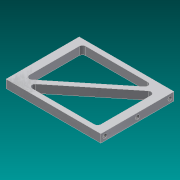
# Autodesk Inventor part: リンク_ふくらはぎ_サブフレーム_1_1(予備案)
Saved by Autodesk Inventor 2016 (Build 200138000, 138)
## iProperties
Created: 2016-06-03
Part Number: リンク_ふくらはぎ_サブフレーム_1_1(予備案)
Material: アルミニウム 2014-T4
Document SubType Name: Modeling
Designer: hiroaki
Density: 2.8 g/cm^3
Appearance: サテン
Mass: 12.9723 g
Surface Area: 43.6812 cm^2
Volume: 4.63295 cm^3
Author: hiroaki
Autodesk Inventor part; units mm, degrees
ref_plane "YZ Plane" through (0, 0, 0) normal (1, 0, 0) x (0, 1, 0)
ref_plane "XZ Plane" through (0, 0, 0) normal (0, 1, 0) x (-1, 0, 0)
ref_plane "XY Plane" through (0, 0, 0) normal (0, 0, 1) x (1, 0, 0)
sketch "スケッチ1" plane through (0, 0, 0) normal (0, 0, 1) x (1, 0, 0)
  line L0 (-29.15, 22.5) -> (29.15, 22.5)
  line L1 (29.15, 22.5) -> (29.15, -22.5)
  line L2 (29.15, -22.5) -> (-29.15, -22.5)
  line L3 (-29.15, -22.5) -> (-29.15, 22.5)
  line L4 (-24.15, 19.5) -> (24.15, 19.5) construction
  line L5 (24.15, 19.5) -> (24.15, -19.5) construction
  line L6 (24.15, -19.5) -> (-24.15, -19.5) construction
  line L7 (-24.15, -19.5) -> (-24.15, 19.5) construction
  line L8 (24.15, 19.5) -> (-24.15, -19.5) construction
  line L9 (-24.15, -17.5721) -> (-24.15, 19.5)
  line L10 (-24.15, 19.5) -> (21.7623, 19.5)
  line L11 (21.7623, 19.5) -> (-24.15, -17.5721)
  line L12 (-21.7623, -19.5) -> (24.15, -19.5)
  line L13 (24.15, -19.5) -> (24.15, 17.5721)
  line L14 (24.15, 17.5721) -> (-21.7623, -19.5)
  line L15 (-29.15, 20) -> (29.15, 20) construction
  line L16 (29.15, -20) -> (-29.15, -20) construction
  line L17 (29.15, 20) -> (29.15, -20) construction
  point P0 (0, 0)
  point P1 (0, 19.5)
  point P2 (0, 22.5)
  point P3 (24.15, 0)
  point P4 (29.15, 0)
  dimension "d0" = 5
  dimension "d1" = 3
  dimension "d2" = 1.5
  dimension "d3" = 40
  dimension "d4" = 2.5
  dimension "d19" = 58.3
  constraints: 36 end point, 6 parallel, 5 collinear, 5 horizontal, 5 midpoint, 4 perpendicular, 4 point on line, 2 horizontal alignment, 2 vertical alignment, 1 vertical, 1 other
  measures "d0" distance between parallel lines of L3 L7
  measures "d1" distance between parallel lines of L0 L4
  measures "d2" distance between parallel lines of L8 L11
  measures "d3" distance between parallel lines of L16 L15
  measures "d4" distance between parallel lines of L2 L16
  measures "d19" distance of L0.start L0.end
extrude "押し出し1" add sketch "スケッチ1" along normal blind 5
sketch "スケッチ2" plane through (29.15, -22.5, 0) normal (1, 0, 0) x (0, 0, -1)
  line L0 (0, 45) -> (-5, 45) projected
  line L1 (-5, 0) -> (-5, 45) projected
  line L2 (0, 22.5) -> (-5, 22.5) construction
  point P0 (-2.5, 2.5)
  point P1 (-2.5, 22.5)
  point P2 (-2.5, 42.5)
  point P3 (-2.5, 45)
  dimension "d7" = 40
  constraints: 3 midpoint, 3 vertical alignment, 2 end point, 1 symmetric about line
  measures "d7" distance of point (-2.5, 42.5) point (-2.5, 2.5)
hole "穴1" at (29.15, -20, 2.5) at (29.15, 0, 2.5) at (29.15, 20, 2.5) direction (-1, 0, 0) diameter 2.459 depth 3 thread size "M3x0.5" class "6H" standard "ISO Metric profile"
mirror "ミラー1" about plane through (0, 0, 0) normal (1, 0, 0) of "穴1"
fillet "フィレット1" radius 2 6 edges at (-21.7623, -19.5, 2.5) (-24.15, -17.5721, 2.5) (24.15, 17.5721, 2.5) (24.15, -19.5, 2.5) (-24.15, 19.5, 2.5) (21.7623, 19.5, 2.5)
equation "\"d3\" = d11_1"
equation "\"d7\" = d3"
equation "\"d11_1\" = 40"
